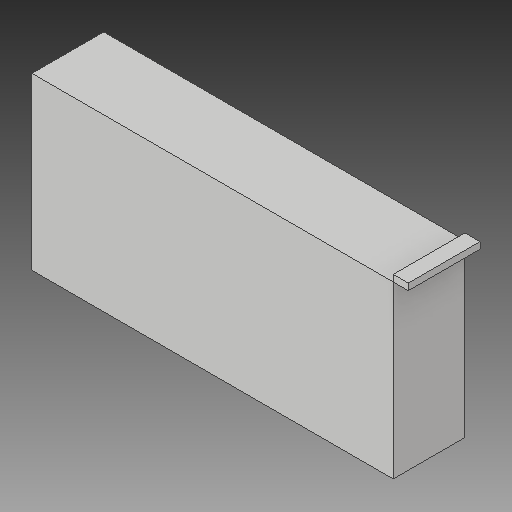
# Autodesk Inventor part: battery
Saved by Autodesk Inventor 2018 (Build 220112000, 112)
## iProperties
Created: 2017-10-09
Part Number: battery
Material: Generic
Document SubType Name: Modeling
Designer: fabre
Density: 1 g/cm^3
Appearance: Default
Author: fabre
Autodesk Inventor part; units mm, degrees
ref_plane "YZ Plane" through (0, 0, 0) normal (1, 0, 0) x (0, 1, 0)
ref_plane "XZ Plane" through (0, 0, 0) normal (0, 1, 0) x (-1, 0, 0)
ref_plane "XY Plane" through (0, 0, 0) normal (0, 0, 1) x (1, 0, 0)
sketch "Sketch1" plane through (0, 0, 0) normal (0, 0, 1) x (1, 0, 0)
  line L0 (0, 0) -> (72, 0)
  line L1 (72, 0) -> (72, 34)
  line L2 (72, 34) -> (0, 34)
  line L3 (0, 34) -> (0, 0)
  line L4 (72, 34) -> (75, 34)
  line L5 (75, 34) -> (75, 35.31)
  line L6 (75, 35.31) -> (72, 35.31)
  line L7 (72, 35.31) -> (72, 34)
  dimension "d0" = 34
  dimension "d1" = 72
  dimension "d2" = 35.31
  dimension "d3" = 75
  constraints: 16 end point, 4 parallel, 2 horizontal, 2 perpendicular
  measures "d0" distance of L2.end L0.start
  measures "d1" distance of L0.start L0.end
  measures "d2" distance between parallel lines of L0 L6
  measures "d3" distance between parallel lines of L3 L5
extrude "Extrusion1" add sketch "Sketch1" along normal blind 14.3
body "Solid1"
